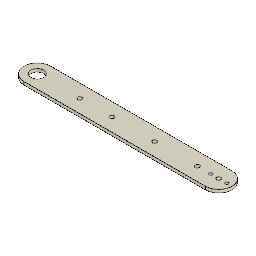
Brazo corto v2 (Autodesk Fusion 360 design; units mm, degrees)
Autodesk Fusion 360 part; units mm, degrees
sketch "Boceto1" plane through (0, 0, 0) normal (0, 0, 1) x (1, 0, 0)
  line L0 (-85, 0) -> (85, 0)
  line L1 (-85, 25) -> (85, 25)
  line L2 (-85, 0) -> (-85, 25) construction
  line L3 (-85, 12.5) -> (85, 12.5) construction
  circle A0 centre (85, 12.5) radius 2
  arc A1 (85, 0) -> (85, 25) centre (85, 12.5) ccw
  arc A2 (-85, 25) -> (-85, 0) centre (-85, 12.5) ccw
  circle A3 centre (-85, 12.5) radius 6
  circle A4 centre (-45, 12.5) radius 2
  circle A5 centre (-15, 12.5) radius 2
  circle A6 centre (25, 12.5) radius 2
  circle A7 centre (65, 12.5) radius 2
  line L4 (85, 12.5) -> (97.5, 12.5) construction
  circle A8 centre (92.5, 12.5) radius 1.5
  circle A9 centre (77.5, 12.5) radius 1.5
  point P0 (-85, 12.5)
  dimension "d1" = 170
  dimension "d2" = 170
  dimension "d3" = 25
  dimension "d5" = 12.5
  dimension "d6" = 4
  dimension "d8" = 12
  dimension "d9" = 4
  dimension "d10" = 40
  dimension "d11" = 4
  dimension "d12" = 4
  dimension "d13" = 30
  dimension "d14" = 40
  dimension "d15" = 4
  dimension "d16" = 40
  dimension "d17" = 3
  dimension "d18" = 7.5
  dimension "d19" = 3
  dimension "d20" = 7.5
  constraint horizontal L0
  constraint midpoint origin L0
  constraint horizontal L1
  constraint coincident L2 P0
  constraint vertical L2
  constraint coincident P0 L3.start
  constraint perpendicular L2 L3
  constraint coincident L3.end A0.centre
  constraint coincident L3 A4.centre
  constraint coincident L3 A5.centre
  constraint coincident L3 A6.centre
  constraint coincident L3 A7.centre
  constraint midpoint A1 L4.end
  constraint coincident L4 A8.centre
  constraint coincident L3 A9.centre
  measures "d1" distance of L0.start L0.end
  measures "d2" distance of L1.start L1.end
  measures "d3" distance of L0 L1
  measures "d5" distance of L0.start P0
  measures "d6" diameter of A0
  measures "d8" diameter of A3
  measures "d9" diameter of A4
  measures "d10" distance of P0 A4.centre
  measures "d11" diameter of A5
  measures "d12" diameter of A6
  measures "d13" distance of A4.centre A5.centre
  measures "d14" distance of A5.centre A6.centre
  measures "d16" distance of A6.centre A7.centre
  measures "d17" diameter of A8
  measures "d18" distance of L3.end A8.centre
  measures "d19" diameter of A9
  measures "d20" distance of L3.end A9.centre
extrude "Extruir1" add sketch "Boceto1" along normal blind 3
